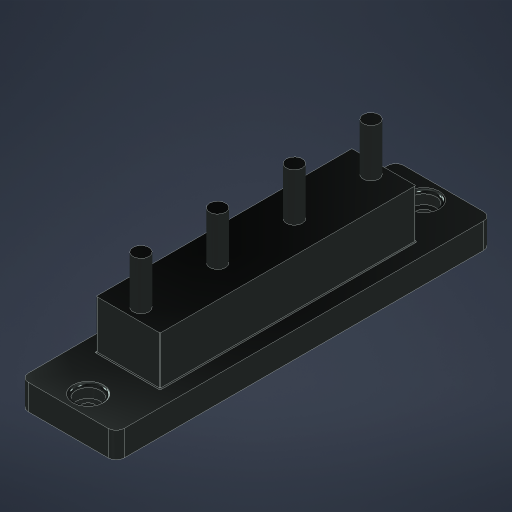
# Autodesk Inventor part: BlueSea_BusBar
Saved by Autodesk Inventor 2023 (Build 270158000, 158)
## iProperties
Created: 2023-01-24
Part Number: BlueSea_BusBar
Material: Generic
Document SubType Name: Modeling
Designer: Nebil
Density: 1 g/cm^3
Appearance: Gunmetal - Polished
Author: Nebil
Autodesk Inventor part; units mm, degrees
ref_plane "YZ Plane" through (0, 0, 0) normal (1, 0, 0) x (0, 1, 0)
ref_plane "XZ Plane" through (0, 0, 0) normal (0, 1, 0) x (-1, 0, 0)
ref_plane "XY Plane" through (0, 0, 0) normal (0, 0, 1) x (1, 0, 0)
sketch "Sketch1" plane through (0, 0, 0) normal (0, 1, 0) x (-1, 0, 0)
  line L0 (-19.05, -74.6125) -> (19.05, -74.6125)
  line L1 (19.05, -74.6125) -> (19.05, 74.6125)
  line L2 (19.05, 74.6125) -> (-19.05, 74.6125)
  line L3 (-19.05, 74.6125) -> (-19.05, -74.6125)
  line L4 (-19.05, -74.6125) -> (19.05, 74.6125) construction
  line L5 (19.05, -74.6125) -> (-19.05, 74.6125) construction
  circle A0 centre (0, 66.675) radius 2.75
  circle A1 centre (0, -66.675) radius 2.75
  line L6 (-12.7, -50.8) -> (12.7, -50.8)
  line L7 (12.7, -50.8) -> (12.7, 50.8)
  line L8 (12.7, 50.8) -> (-12.7, 50.8)
  line L9 (-12.7, 50.8) -> (-12.7, -50.8)
  line L10 (-12.7, -50.8) -> (12.7, 50.8) construction
  line L11 (12.7, -50.8) -> (-12.7, 50.8) construction
  circle A2 centre (0, -15.24) radius 3.175
  circle A3 centre (0, -45.72) radius 3.175
  circle A4 centre (0, 15.24) radius 3.175
  circle A5 centre (0, 45.72) radius 3.175
  point P0 (0, 0)
  point P1 (0, 50.8)
  dimension "d0" = 38.1
  dimension "d1" = 149.225
  dimension "d2" = 133.35
  dimension "d3" = 5.5
  dimension "d4" = 5.5
  dimension "d7" = 25.4
  dimension "d8" = 101.6
  dimension "d9" = 6.35
  dimension "d10" = 6.35
  dimension "d11" = 6.35
  dimension "d12" = 6.35
  dimension "d13" = 30.48
  dimension "d14" = 30.48
  dimension "d16" = 5.08
  dimension "d17" = 5.08
  dimension "d19" = 30.48
  dimension "d20" = 66.675
  constraints: 24 end point, 6 centre point, 6 vertical alignment, 5 midpoint, 4 parallel, 2 horizontal, 2 perpendicular
  measures "d0" distance of L2.end L1.end
  measures "d1" distance of L1.end L0.end
  measures "d2" distance of A1.centre A0.centre
  measures "d3" diameter of A0
  measures "d4" diameter of A1
  measures "d7" distance of L8.end L7.end
  measures "d8" distance of L6.end L7.end
  measures "d9" diameter of A5
  measures "d10" diameter of A4
  measures "d11" diameter of A2
  measures "d12" diameter of A3
  measures "d13" distance of A3.centre A2.centre
  measures "d14" distance of A4.centre A5.centre
  measures "d16" distance from line of L6 A3.centre
  measures "d17" distance of point (0, 50.8) A5.centre
  measures "d19" distance of A2.centre A4.centre
  measures "d20" distance of A1.centre point (0, 0)
extrude "Extrusion1" add sketch "Sketch1" along normal blind 10.16 contours L3 L2 L1 L0 | L9 L8 L7 L6 | A2 | A3 | A4 | A5
extrude "Extrusion2" add sketch "Sketch1" along normal blind 29.464 contours L9 L8 L7 L6
extrude "Extrusion3" add sketch "Sketch1" along normal blind 48.514 contours A2 | A3 | A4 | A5
sketch "Sketch2" plane through (0, 10.16, 0) normal (0, 1, 0) x (1, 0, 0)
  circle A0 centre (0, -66.675) radius 4.875
  circle A1 centre (0, -66.675) radius 2.75 projected
  circle A2 centre (0, 66.675) radius 4.875
  circle A3 centre (0, 66.675) radius 2.75 projected
  point P0 (0, 0)
  dimension "d25" = 9.75
  dimension "d26" = 9.75
  constraints: 2 centre point, 2 concentric
  measures "d25" diameter of A0
  measures "d26" diameter of A2
extrude "Extrusion4" cut sketch "Sketch2" against normal blind 5 contours A0 | A2 | A3
fillet "Fillet1" radius 0.3175 8 edges at (12.7, 19.812, 50.8) (-12.7, 19.812, 50.8) (12.7, 19.812, -50.8) (-12.7, 19.812, -50.8) (12.7, 10.16, 0) (0, 10.16, 50.8) (-12.7, 10.16, 0) (0, 10.16, -50.8)
fillet "Fillet2" radius 3.175 4 edges at (19.05, 5.08, 74.6125) (-19.05, 5.08, 74.6125) (19.05, 5.08, -74.6125) (-19.05, 5.08, -74.6125)
fillet "Fillet3" radius 1.27 2 edges at (-4.875, 10.16, 66.675) (-4.875, 10.16, -66.675)
equation "\"d4\" = d3"
equation "\"d10\" = d9"
equation "\"d11\" = d9"
equation "\"d12\" = d9"
equation "\"d20\" = 0.5 * d2"
body "Solid1"
